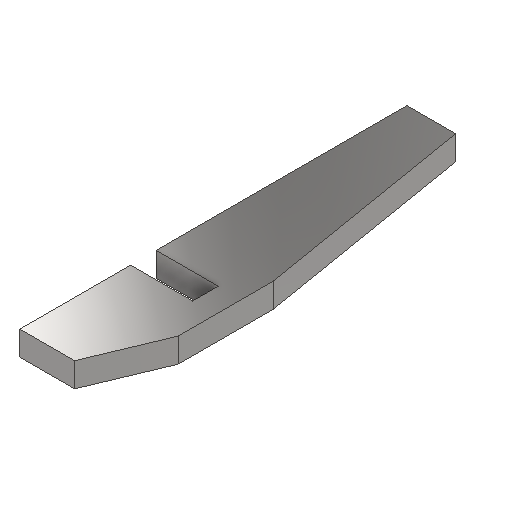
# Autodesk Inventor part: Feather_0_aerofoil_frame_support_p2
Saved by Autodesk Inventor 2022 (Build 260153000, 153)
## iProperties
Created: 2022-09-03
Part Number: Feather_0_aerofoil_frame_support_p2
Material: Iron, Malleable
Document SubType Name: Modeling
Designer: dell
Density: 7.15 g/cm^3
Appearance: Semi-Polished
Author: dell
Autodesk Inventor part; units mm, degrees
ref_plane "YZ Plane" through (0, 0, 0) normal (1, 0, 0) x (0, 1, 0)
ref_plane "XZ Plane" through (0, 0, 0) normal (0, 1, 0) x (-1, 0, 0)
ref_plane "XY Plane" through (0, 0, 0) normal (0, 0, 1) x (1, 0, 0)
sketch "Sketch1" plane through (0, 0, 0) normal (0, 1, 0) x (-1, 0, 0)
  line L0 (0, 0) -> (7, 0)
  line L1 (7, 0) -> (7, -31.8)
  line L2 (7, -31.8) -> (0, -31.8)
  line L3 (0, -31.8) -> (0, 0)
  line L4 (7, -9.1) -> (1.9, -9.1)
  line L5 (1.9, -9.1) -> (1.9, -11.2)
  line L6 (1.9, -11.2) -> (7, -11.2)
  line L7 (7, -11.2) -> (7, -9.1)
  point P0 (7, -11.2)
  dimension "d0" = 7
  dimension "d1" = 31.8
  dimension "d2" = 2.1
  dimension "d3" = 5.1
  dimension "d4" = 9.1
  constraints: 16 end point, 4 parallel, 2 horizontal, 2 perpendicular, 1 point on line
  measures "d0" distance between parallel lines of L3 L1
  measures "d1" distance between parallel lines of L2 L0
  measures "d2" distance of L4.end L5.end
  measures "d3" distance between parallel lines of L1 L5
  measures "d4" distance between parallel lines of L0 L4
extrude "Extrusion1" add sketch "Sketch1" along normal blind 2 contours L0 L1 L4 L5 L6 L2 L3
chamfer "Chamfer1" distance 2.5 distance2 6 1 edges at (0, 1, 0) measured on face at (-0.5, 1, 0)
chamfer "Chamfer2" distance 18 distance2 3 1 edges at (0, 1, -31.8) measured on face at (0, 1, -31.3)
body "Solid1"
